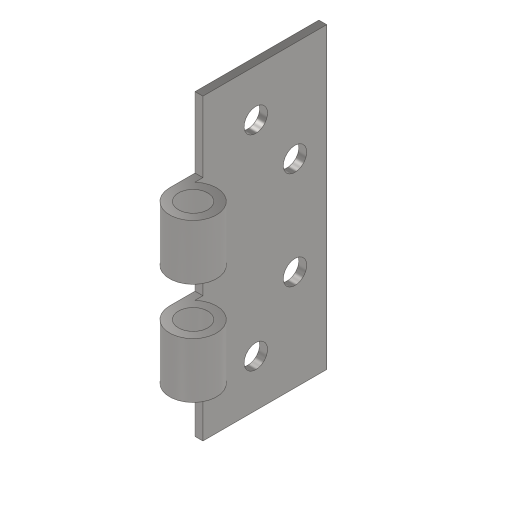
# Autodesk Inventor part: zawias-prawy
Saved by Autodesk Inventor 2023.2 (Build 272271000, 271)
## iProperties
Created: 2022-12-05
Part Number: zawias-prawy
Material: Stainless Steel
Document SubType Name: Modeling
Designer: GUT
Mass: 53.8004 g
Surface Area: 72.4388 cm^2
Volume: 6.72505 cm^3
Density: 8 g/cm^3
Appearance: Semi-Polished
Author: GUT
Autodesk Inventor part; units mm, degrees
ref_plane "YZ Plane" through (0, 0, 0) normal (1, 0, 0) x (0, 1, 0)
ref_plane "XZ Plane" through (0, 0, 0) normal (0, 1, 0) x (-1, 0, 0)
sketch "Sketch1" plane through (0, 0, 0) normal (1, 0, 0) x (0, 1, 0)
  line L0 (7.182, 51.3195) -> (83.382, 51.3195)
  line L1 (83.382, 51.3195) -> (83.382, 13.2195)
  line L2 (83.382, 13.2195) -> (7.182, 13.2195)
  line L3 (7.182, 13.2195) -> (7.182, 51.3195)
  line L4 (39.282, 51.3195) -> (51.282, 51.3195)
  line L5 (51.282, 51.3195) -> (51.282, 44.8195)
  line L6 (51.282, 44.8195) -> (39.282, 44.8195)
  line L7 (39.282, 44.8195) -> (39.282, 51.3195)
  line L8 (45.282, 13.2195) -> (45.282, 51.3195) construction
  line L9 (83.382, 44.8195) -> (65.382, 44.8195)
  line L10 (65.382, 44.8195) -> (65.382, 51.3195)
  line L11 (65.382, 51.3195) -> (83.382, 51.3195)
  line L12 (83.382, 51.3195) -> (83.382, 44.8195)
  line L13 (7.182, 51.3195) -> (25.182, 51.3195)
  line L14 (25.182, 51.3195) -> (25.182, 44.8195)
  line L15 (25.182, 44.8195) -> (7.182, 44.8195)
  line L16 (7.182, 44.8195) -> (7.182, 51.3195)
  circle A0 centre (71.382, 31.3195) radius 3
  circle A1 centre (57.782, 21.3195) radius 3
  circle A2 centre (19.182, 31.3195) radius 3
  circle A3 centre (32.782, 21.3195) radius 3
  point P0 (0, 0)
  point P1 (7.182, 44.8195)
  dimension "d0" = 38.1
  dimension "d1" = 76.2
  dimension "d2" = 12
  dimension "d3" = 6.5
  dimension "d4" = 18
  dimension "d7" = 6
  dimension "d8" = 6
  dimension "d9" = 20
  dimension "d10" = 30
  dimension "d11" = 12.5
  dimension "d12" = 26.1
  constraints: 34 end point, 8 parallel, 4 centre point, 4 horizontal, 4 perpendicular, 3 equal length, 3 point on line, 2 midpoint, 2 symmetric about line, 3 other
  measures "d0" distance of L0.end L1.end
  measures "d1" distance of L1.end L2.end
  measures "d2" distance of L5.end L6.end
  measures "d3" distance of L4.end L5.end
  measures "d4" distance of L9.start L9.end
  measures "d7" diameter of A0
  measures "d8" diameter of A1
  measures "d9" distance from line of L0 A0.centre
  measures "d10" distance from line of L0 A1.centre
  measures "d11" distance from line of L8 A1.centre
  measures "d12" distance from line of L8 A0.centre
extrude "Extrusion1" add sketch "Sketch1" along normal blind 2 contours L0 L7 L6 L5 L10 L9 L1 L2 L3 L15 L14
ref_plane "Work Plane1" through (2, 45.282, 44.8195) normal (0, -1, 0) x (1, 0, 0)
sketch "Sketch2" plane through (0, 65.382, 51.3195) normal (0, 1, 0) x (1, 0, 0)
  line L0 (0, 6.5) -> (0, 0) projected
  line L1 (0, 0) -> (2, 0) projected
  line L2 (2, 6.5) -> (2, 0) projected
  line L3 (0, 6.5) -> (2, 6.5) projected
  circle A0 centre (6, 0) radius 6
  circle A1 centre (6, 0) radius 3.75
  point P0 (0, 51.3195)
  point P1 (2, 4.4721)
  dimension "d13" = 12
  dimension "d14" = 7.5
  dimension "d15" = 4
  constraints: 2 centre point, 1 coincident
  measures "d13" diameter of A0
  measures "d14" diameter of A1
  measures "d15" distance from line of L2 A1.centre
extrude "Extrusion2" add sketch "Sketch2" against normal up to surface (14.1 mm away) contours L1 L2 A0 picked at (11.1556, -0.7778)
mirror "Mirror1" about plane through (2, 45.282, 44.8195) normal (0, -1, 0) of "Extrusion2"
equation "\"d8\" = d7"
body "Solid1"
